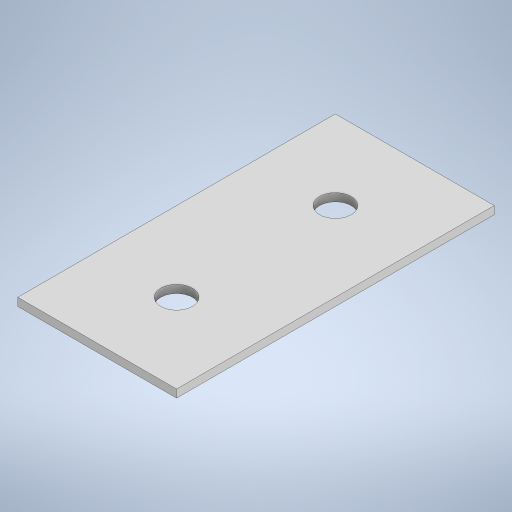
# Autodesk Inventor part: Соединитель 40х80
Saved by Autodesk Inventor 2023 (Build 270158000, 158)
## iProperties
Created: 2022-05-05
Part Number: Соединитель 40х80
Material: Типовые
Document SubType Name: Modeling
Designer: avkap
Density: 1 g/cm^3
Appearance: По умолчанию
Author: avkap
Autodesk Inventor part; units mm, degrees
ref_plane "YZ Plane" through (0, 0, 0) normal (1, 0, 0) x (0, 1, 0)
ref_plane "XZ Plane" through (0, 0, 0) normal (0, 1, 0) x (-1, 0, 0)
ref_plane "XY Plane" through (0, 0, 0) normal (0, 0, 1) x (1, 0, 0)
sketch "Эскиз1" plane through (0, 0, 0) normal (0, 1, 0) x (-1, 0, 0)
  line L0 (0, 0) -> (-40, 0)
  line L1 (-40, 0) -> (-40, -80)
  line L2 (-40, -80) -> (0, -80)
  line L3 (0, -80) -> (0, 0)
  line L4 (-20, 0) -> (-20, -20)
  line L5 (-20, -20) -> (-20, -60)
  circle A0 centre (-20, -20) radius 4
  circle A1 centre (-20, -60) radius 4
  dimension "d0" = 40
  dimension "d1" = 80
  dimension "d2" = 20
  dimension "d3" = 40
  dimension "d4" = 8
  dimension "d5" = 8
  constraints: 12 end point, 2 centre point, 2 coincident, 2 parallel, 1 horizontal, 1 midpoint, 1 perpendicular, 1 point on line, 1 vertical
  measures "d0" distance of L2.end L1.end
  measures "d1" distance of L1.end L0.end
  measures "d2" distance of L4.start L4.end
  measures "d3" distance of L4.end L5.end
  measures "d4" diameter of A0
  measures "d5" diameter of A1
extrude "Выдавливание1" add sketch "Эскиз1" along normal blind 2
